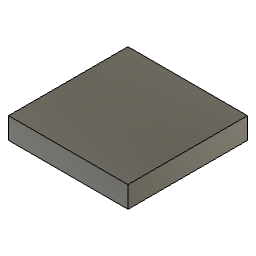
box v1 (Autodesk Fusion 360 design; units mm, degrees)
Autodesk Fusion 360 part; units mm, degrees
sketch "Sketch1" plane through (0, 0, 0) normal (0, 1, 0) x (1, 0, 0)
  line L0 (47.5, 47.5) -> (-47.5, 47.5)
  line L1 (-47.5, 47.5) -> (-47.5, -47.5)
  line L2 (-47.5, -47.5) -> (47.5, -47.5)
  line L3 (47.5, -47.5) -> (47.5, 47.5)
  line L4 (47.5, 47.5) -> (-47.5, -47.5) construction
  line L5 (-47.5, 47.5) -> (47.5, -47.5) construction
  dimension "d8" = 95
  dimension "d9" = 95
  constraint horizontal L0
  constraint perpendicular L0 L1
  constraint parallel L0 L2
  constraint parallel L1 L3
  constraint coincident L4 origin
  constraint coincident L5 origin
  measures "d8" distance of L1.end L2.end
  measures "d9" distance of L0.end L1.end
box "BoxPrimitive1" add length 95 width 95 height 17 placed x (0, 1, 0) y (-1, 0, 0) z (0, 0, 1) at (1.0639, 0, 0)
